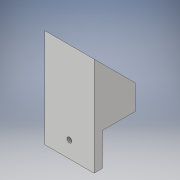
# Autodesk Inventor part: spiegelhalter
Saved by Autodesk Inventor 2017 (Build 210142000, 142)
## iProperties
Part Number: spiegelhalter
Material: Generisch
Document SubType Name: Modeling
Designer: Fabio
Density: 1 g/cm^3
Appearance: Vorgabe
Author: Fabio
Autodesk Inventor part; units mm, degrees
ref_plane "YZ Plane" through (0, 0, 0) normal (1, 0, 0) x (0, 1, 0)
ref_plane "XZ Plane" through (0, 0, 0) normal (0, 1, 0) x (-1, 0, 0)
ref_plane "XY Plane" through (0, 0, 0) normal (0, 0, 1) x (1, 0, 0)
sketch "Skizze1" plane through (0, 0, 0) normal (1, 0, 0) x (0, 1, 0)
  line L0 (0, 0) -> (0, -40)
  line L1 (0, -40) -> (40, -40)
  line L2 (40, -40) -> (0, 0)
  dimension "d0" = 45
  dimension "d1" = 40
  constraints: 6 end point, 1 perpendicular, 1 vertical
  measures "d0" angle of L0 L2
  measures "d1" distance of L0.end L1.end
extrude "Extrusion1" add sketch "Skizze1" along normal blind 30
sketch "Skizze4" plane through (0, 0, -40) normal (0, 0, -1) x (-1, 0, 0)
  line L0 (-30, 0) -> (-30, 40) projected
  line L1 (0, 0) -> (-30, 0)
  line L2 (-30, 0) -> (-30, 5)
  line L3 (-30, 5) -> (0, 5)
  line L4 (0, 5) -> (0, 0)
  dimension "d19" = 5
  constraints: 8 end point, 2 parallel, 1 horizontal, 1 perpendicular, 1 point on line
  measures "d19" distance of L1.end L2.end
extrude "Extrusion2" add sketch "Skizze4" along normal blind 20
sketch "Skizze5" plane through (0, 5, -40) normal (0, 1, 0) x (1, 0, 0)
  line L0 (30, 20) -> (0, 20) construction
  line L1 (15, 20) -> (15, 0) construction
  line L2 (0, 0) -> (30, 0) construction
  line L3 (0, 0) -> (0, 20) construction
  line L4 (30, 0) -> (0, 0) construction
  line L5 (30, 0) -> (30, 20) construction
  line L6 (0, 20) -> (30, 20) construction
  line L7 (0, 0) -> (0, 20) construction
  line L8 (0, 10) -> (30, 10) construction
  point P0 (0, -40)
  point P1 (15, 10)
  constraints: 5 midpoint, 4 end point
hole "Bohrung2" at (15, 5, -50) direction (0, -1, 0) diameter 3 end through all
sketch "Skizze6" plane through (30, 0, 0) normal (1, 0, 0) x (0, 0, -1)
  line L0 (40, 5) -> (40, 40) projected
  line L1 (40, 40) -> (20, 40)
  line L2 (20, 40) -> (20, 25)
  line L3 (20, 25) -> (40, 25)
  line L4 (40, 25) -> (40, 40)
  point P0 (0, 0)
  dimension "d29" = 15
  dimension "d30" = 20
  constraints: 8 end point, 2 parallel, 1 horizontal, 1 perpendicular
  measures "d29" distance of L1.end L2.end
  measures "d30" distance of L2.end L3.end
extrude "Extrusion3" cut sketch "Skizze6" against normal through all
